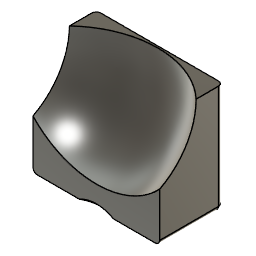
Backpack (Autodesk Fusion 360 design; units mm, degrees)
Autodesk Fusion 360 part; units mm, degrees
sketch "Sketch15" plane through (0, 0, 0) normal (0, 1, 0) x (1, 0, 0)
  line L0 (0, 0) -> (-140, 0)
  line L1 (-140, 0) -> (-140, 120)
  line L2 (-140, 120) -> (0, 120)
  line L3 (0, 120) -> (0, 0)
  line L4 (0, 0) -> (-70, 0) construction
  line L5 (-70, 0) -> (-70, 102) construction
  line L6 (-70, 102) -> (-70, 153) construction
  line L7 (-70, 120) -> (-70, 0)
  arc A0 (-108.8844, 120) -> (-70, 102) centre (-70, 153) ccw
  arc A1 (-70, 102) -> (-140, 74.1889) centre (-70, 0) ccw
  dimension "d65" = 140
  dimension "d66" = 120
  dimension "d67" = 70
  dimension "d68" = 102
  dimension "d69" = 204
  dimension "d70" = 51
  dimension "d71" = 102
  constraint horizontal L0
  constraint vertical L1
  constraint horizontal L2
  constraint vertical L3
  constraint coincident L0.start L3.end
  constraint perpendicular L1 L4
  constraint perpendicular L4 L5
  constraint coincident L4.end L5.start
  constraint perpendicular L2 L6
  constraint coincident L6.end A0.centre
  constraint midpoint L2 L7.start
  constraint coincident L2 A0.start
  constraint coincident L1 A1.end
  measures "d65" distance of L0.start L0.end
  measures "d66" distance of L0.end L1.end
  measures "d67" distance of L0.start L4.end
  measures "d68" distance of L4.end L5.end
  measures "d69" diameter of A1
  measures "d70" distance of L5.end L6.end
  measures "d71" diameter of A0
extrude "Extrude9" add sketch "Sketch15" along normal blind 70
ref_plane "WorkPlane3" through (-70, -34, -60) normal (0, 1, 0) x (0, 0, 1)
sketch "Sketch16" plane through (0, -34, 0) normal (0, 1, 0) x (1, 0, 0)
  line L0 (0, 0) -> (-70, 0) construction
  line L1 (-70, 0) -> (-70, 153) construction
  line L2 (-70, 0) -> (-70, 204)
  line L3 (-70, 0) -> (-172, 0)
  arc A0 (-70, 102) -> (-172, 0) centre (-70, 0) ccw
  arc A1 (-70, 204) -> (-70, 102) centre (-70, 153) ccw
  dimension "d75" = 70
  dimension "d76" = 153
  dimension "d77" = 204
  dimension "d78" = 102
  constraint coincident L0.start origin
  constraint horizontal L0
  constraint perpendicular L0 L1
  constraint coincident L0.end L1.start
  constraint coincident L1.end A1.centre
  constraint parallel L1 L2
  constraint perpendicular L1 L3
  constraint coincident L1 A0.start
  measures "d75" distance of L0.start L0.end
  measures "d76" distance of L0.end L1.end
  measures "d77" diameter of A0
  measures "d78" diameter of A1
revolve "Revolve6" cut sketch "Sketch16" angle 360 about axis through (-70, -34, 0) along (0, 0, -1)
fillet "Fillet1" radius 5 1 edges at (-70, 70, -120)
fillet "Fillet2" radius 5 3 edges at (-140, 32.5, -120) (-140, 68.5355, -118.5355) (-140, 70, -57.5)
fillet "Fillet3" radius 5 3 edges at (0, 32.5, -120) (0, 68.5355, -118.5355) (0, 70, -57.5)
